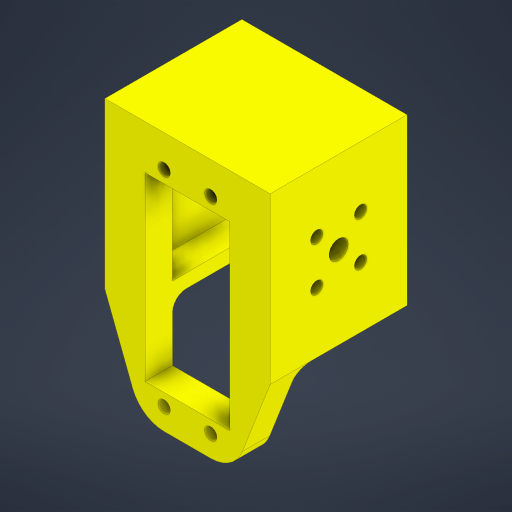
# Autodesk Inventor part: Servo-house
Saved by Autodesk Inventor 2023 (Build 270158000, 158)
## iProperties
Created: 2023-08-17
Part Number: Servo-house
Material: PBT Plastic
Document SubType Name: Modeling
Designer: Abhinav
Density: 1.31 g/cm^3
Appearance: Default(1)
Mass: 91.1273 g
Surface Area: 272.762 cm^2
Volume: 69.5628 cm^3
Author: Abhinav
Autodesk Inventor part; units mm, degrees
ref_plane "YZ Plane" through (0, 0, 0) normal (1, 0, 0) x (0, 1, 0)
ref_plane "XZ Plane" through (0, 0, 0) normal (0, 1, 0) x (-1, 0, 0)
ref_plane "XY Plane" through (0, 0, 0) normal (0, 0, 1) x (1, 0, 0)
sketch "Sketch1" plane through (0, 0, 0) normal (0, 0, 1) x (1, 0, 0)
  line L0 (-25.15, 25.15) -> (25.15, 25.15)
  line L1 (25.15, 25.15) -> (25.15, -25.15)
  line L2 (25.15, -25.15) -> (-25.15, -25.15)
  line L3 (-25.15, -25.15) -> (-25.15, 25.15)
  line L4 (-25.15, 25.15) -> (25.15, -25.15) construction
  line L5 (25.15, 25.15) -> (-25.15, -25.15) construction
  line L6 (-30.15, 30.15) -> (30.15, 30.15)
  line L7 (30.15, 30.15) -> (30.15, -30.15)
  line L8 (30.15, -30.15) -> (-30.15, -30.15)
  line L9 (-30.15, -30.15) -> (-30.15, 30.15)
  line L10 (-30.15, 30.15) -> (30.15, -30.15) construction
  line L11 (30.15, 30.15) -> (-30.15, -30.15) construction
  line L12 (0, 25.15) -> (0, 18.5) construction
  line L13 (0, 18.5) -> (8.5, 18.5) construction
  circle A0 centre (8.5, 18.5) radius 2.25
  line L14 (8.5, 18.5) -> (-8.5, 18.5)
  line L15 (-8.5, 18.5) -> (-8.5, -56.5)
  line L16 (-8.5, -56.5) -> (8.5, -56.5)
  line L17 (8.5, -56.5) -> (8.5, 18.5)
  circle A1 centre (8.5, -56.5) radius 2.25
  line L18 (-8.5, 18.5) -> (8.5, -56.5) construction
  line L19 (-15.5, 14) -> (15.5, 14)
  line L20 (15.5, 14) -> (15.5, -52)
  line L21 (15.5, -52) -> (-15.5, -52)
  line L22 (-15.5, -52) -> (-15.5, 14)
  line L23 (-15.5, 14) -> (15.5, -52) construction
  line L24 (15.5, 14) -> (-15.5, -52) construction
  circle A2 centre (-8.5, -56.5) radius 2.25
  circle A3 centre (-8.5, 18.5) radius 2.25
  line L25 (-30.15, -30.15) -> (-20.0032, -56.4398)
  arc A4 (-20.0032, -56.4398) -> (-8.5, -64.3302) centre (-8.5, -52) ccw
  line L26 (0, 0) -> (0, -19) construction
  line L27 (30.15, -30.15) -> (20.0032, -56.4398)
  line L28 (-8.5, -64.3302) -> (8.5, -64.3302)
  arc A5 (8.5, -64.3302) -> (20.0032, -56.4398) centre (8.5, -52) ccw
  point P0 (15.5, -25.15)
  point P1 (15.5, -30.15)
  point P2 (-15.5, -30.15)
  point P3 (-15.5, -25.15)
  dimension "d0" = 50.3
  dimension "d2" = 60.3
  dimension "d4" = 6.65
  dimension "d5" = 8.5
  dimension "d6" = 4.5
  dimension "d7" = 17
  dimension "d8" = 75
  dimension "d10" = 31
  dimension "d11" = 66
  constraints: 58 end point, 8 midpoint, 8 parallel, 7 perpendicular, 6 centre point, 4 coincident, 4 horizontal, 4 point on circle, 3 equal radius, 3 point on line, 2 symmetric about line, 2 tangent, 1 vertical
  measures "d0" distance of L1.end L2.end
  measures "d2" distance of L7.end L8.end
  measures "d4" distance of L12.start L12.end
  measures "d5" distance of L12.end L13.end
  measures "d6" diameter of A0
  measures "d7" distance of L16.end L15.end
  measures "d8" distance of L15.end L14.end
  measures "d10" distance of L20.end L21.end
  measures "d11" distance of L19.end L20.end
extrude "Extrusion1" add sketch "Sketch1" against normal blind 40 contours L3 L2 L22 L8 L9 L6 L7 L20 L1 L0
extrude "Extrusion2" add sketch "Sketch1" along normal blind 10 contours L3 L2 L22 L8 L9 L6 L7 L20 L1 L0 | L0 L1 L2 L20 L19 L17 A0 L14 A3 L15 L22 L3 | L22 L21 L15 A2 L16 A1 L17 L20 L8 L27 A5 L28 A4 L25 | L15 A3 L14 A0 L17 L19 | L21 L17 A1 L16 A2 L15
fillet "Fillet1" radius 5 2 edges at (22.825, -30.15, 0) (-22.825, -30.15, 0)
sketch "Sketch2" plane through (30.15, -30.15, -40) normal (1, 0, 0) x (0, 0, -1)
  line L0 (0, 60.3) -> (0, 0) projected
  line L1 (-10, 60.3) -> (-40, 60.3)
  line L2 (-40, 60.3) -> (-40, 0)
  line L3 (-40, 0) -> (-10, 0)
  line L4 (-10, 0) -> (-10, 60.3)
  line L5 (-35, 0) -> (0, 0) construction
  circle A0 centre (-25, 30.15) radius 3.5
  line L6 (0.0184, 0) -> (-9.9816, 0) construction
  line L7 (-35, 0) -> (0, 0) projected
  line L8 (-33, 38.15) -> (-17, 38.15) construction
  line L9 (-17, 38.15) -> (-17, 22.15) construction
  line L10 (-17, 22.15) -> (-33, 22.15) construction
  line L11 (-33, 22.15) -> (-33, 38.15) construction
  line L12 (-33, 38.15) -> (-17, 22.15) construction
  line L13 (-17, 38.15) -> (-33, 22.15) construction
  circle A1 centre (-33, 38.15) radius 2.25
  circle A2 centre (-17, 38.15) radius 2.25
  circle A3 centre (-17, 22.15) radius 2.25
  circle A4 centre (-33, 22.15) radius 2.25
  line L14 (-25, 30.15) -> (-20.3356, 34.8144) construction
  line L15 (-10, 60.3) -> (-40, 0) construction
  line L16 (-25, 30.15) -> (-30.0486, 30.15) construction
  point P0 (-40, 30.15)
  dimension "d20" = 30
  dimension "d21" = 7
  dimension "d24" = 10
  dimension "d25" = 16
  dimension "d27" = 4.5
  dimension "d28" = 60.3
  constraints: 28 end point, 5 centre point, 4 coincident, 4 parallel, 3 equal radius, 3 horizontal, 3 midpoint, 3 perpendicular, 1 point on line, 1 other
  measures "d20" distance of L3.end L2.end
  measures "d21" diameter of A0
  measures "d24" distance of L6.start L6.end
  measures "d25" distance of L9.end L10.end
  measures "d27" diameter of A1
  measures "d28" distance of L1.end L2.end
extrude "Extrusion3" cut sketch "Sketch2" against normal blind 65 contours A0 | A1 | A2 | A3 | A4
body "Solid1"
